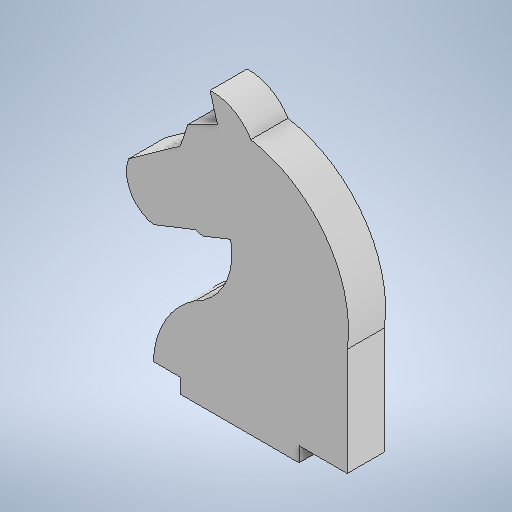
# Autodesk Inventor part: KIGTH TOP 1.0
Saved by Autodesk Inventor 2025.1 (Build 291241000, 241)
## iProperties
Created: 2024-10-24
Part Number: KIGTH TOP 1.0
Material: Genérico
Document SubType Name: Modeling
Designer: Octavio
Density: 1 g/cm^3
Appearance: Valor por defecto
Author: Octavio
Autodesk Inventor part; units mm, degrees
ref_plane "YZ Plane" through (0, 0, 0) normal (1, 0, 0) x (0, 1, 0)
ref_plane "XZ Plane" through (0, 0, 0) normal (0, 1, 0) x (-1, 0, 0)
ref_plane "XY Plane" through (0, 0, 0) normal (0, 0, 1) x (1, 0, 0)
sketch "Boceto1" plane through (0, 0, 0) normal (0, 0, 1) x (1, 0, 0)
  line L0 (-70.4693, 87.7725) -> (72.3878, 87.7725) construction
  line L1 (72.3878, 87.7725) -> (72.3878, -52.7037) construction
  line L2 (72.3878, -52.7037) -> (-70.4693, -52.7037) construction
  line L3 (-70.4693, -52.7037) -> (-70.4693, 87.7725) construction
  line L4 (-16, 0) -> (16, 0)
  line L5 (16, 0) -> (16, 4)
  line L6 (16, 4) -> (29, 4)
  line L7 (29, 4) -> (29, 33)
  arc A0 (29, 33) -> (3, 69) centre (-2.439, 37.6829) ccw
  arc A1 (3, 69) -> (-8, 75) centre (-7.5, 62.8333) ccw
  line L8 (-8, 75) -> (-6, 68)
  line L9 (-6, 68) -> (-14, 64)
  line L10 (-14, 64) -> (-16, 58)
  line L11 (-16, 58) -> (-30, 48)
  arc A2 (-30, 48) -> (-23.3333, 36) centre (-21.5351, 44.8509) ccw
  line L12 (-23.3333, 36) -> (-12, 40.4647)
  line L13 (-12, 40.4647) -> (-10, 40)
  line L14 (-10, 40) -> (-2.439, 42.9786)
  arc A3 (-12, 23.8479) -> (-2.439, 42.9786) centre (-19.6735, 39.6374) ccw
  arc A4 (-12, 23.8479) -> (-23.3333, 4) centre (1.7175, 2.8554) ccw
  line L15 (-23.3333, 4) -> (-16, 4)
  line L16 (-16, 4) -> (-16, 0)
  point P0 (0, 0)
  constraints: 26 end point, 10 point on circle, 5 centre point, 4 perpendicular, 2 horizontal, 1 parallel, 2 other
extrude "Extrusión1" add sketch "Boceto1" along normal mid plane 10
